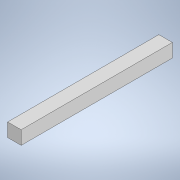
# Autodesk Inventor part: Connector
Saved by Autodesk Inventor 2020.1 (Build 241239000, 239)
## iProperties
Created: 2020-02-13
Part Number: Connector
Material: Generic
Document SubType Name: Modeling
Designer: super
Density: 1 g/cm^3
Appearance: Default
Author: super
Autodesk Inventor part; units mm, degrees
ref_plane "YZ Plane" through (0, 0, 0) normal (1, 0, 0) x (0, 1, 0)
ref_plane "XZ Plane" through (0, 0, 0) normal (0, 1, 0) x (-1, 0, 0)
ref_plane "XY Plane" through (0, 0, 0) normal (0, 0, 1) x (1, 0, 0)
sketch "Sketch1" plane through (0, 0, 0) normal (0, 1, 0) x (-1, 0, 0)
  line L0 (0, 0) -> (6.35, 0)
  line L1 (6.35, 0) -> (6.35, -70)
  line L2 (6.35, -70) -> (0, -70)
  line L3 (0, -70) -> (0, 0)
  dimension "d0" = 6.35
  dimension "d1" = 70
  constraints: 8 end point, 2 perpendicular, 1 horizontal, 1 parallel
  measures "d0" distance of L0.start L0.end
  measures "d1" distance of L0.end L1.end
extrude "Extrusion1" add sketch "Sketch1" along normal blind 6.35
sketch "Sketch2" plane through (0, 6.35, 0) normal (0, 1, 0) x (1, 0, 0)
  line L0 (0, 0) -> (0, 70) projected
  line L1 (0, 0) -> (0, -1)
  line L2 (0, -1) -> (-6.35, -1)
  line L3 (-6.35, -1) -> (-6.35, 0)
  line L4 (-6.35, 0) -> (0, 0) projected
  line L5 (-6.35, 0) -> (0, 0)
  dimension "d4" = 1
  constraints: 8 end point, 3 perpendicular, 1 vertical
  measures "d4" distance of L0.start L1.end
extrude "Extrusion2" add sketch "Sketch2" against normal blind 6.35
body "Solid1"
